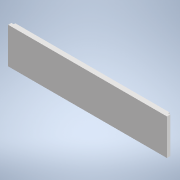
# Autodesk Inventor part: Arcade_FrontBottom
Saved by Autodesk Inventor 2022 (Build 260153000, 153)
## iProperties
Created: 2023-12-22
Part Number: Arcade_FrontBottom
Material: Generic
Document SubType Name: Modeling
Designer: Petr Černý
Density: 1 g/cm^3
Appearance: Default
Author: Petr Černý
Autodesk Inventor part; units mm, degrees
ref_plane "YZ Plane" through (0, 0, 0) normal (1, 0, 0) x (0, 1, 0)
ref_plane "XZ Plane" through (0, 0, 0) normal (0, 1, 0) x (-1, 0, 0)
ref_plane "XY Plane" through (0, 0, 0) normal (0, 0, 1) x (1, 0, 0)
sketch "Sketch1" plane through (0, 0, 0) normal (0, 0, 1) x (1, 0, 0)
  line L0 (-46.7038, 15.5679) -> (443.2962, 15.5679)
  line L1 (443.2962, 15.5679) -> (443.2962, -95.4321)
  line L2 (443.2962, -95.4321) -> (-46.7038, -95.4321)
  line L3 (-46.7038, -95.4321) -> (-46.7038, 15.5679)
  point P0 (0, 0)
  dimension "d0" = 490
  dimension "d1" = 111
  constraints: 8 end point, 2 parallel, 1 horizontal, 1 perpendicular
  measures "d0" distance of L1.end L2.end
  measures "d1" distance of L0.end L1.end
extrude "Extrusion1" add sketch "Sketch1" along normal blind 15
sketch "Sketch2" plane through (443.2962, -95.4321, 0) normal (1, 0, 0) x (0, 0, -1)
  line L0 (0, 0) -> (0, 111) projected
  line L1 (0, 111) -> (-5, 111)
  line L2 (-5, 111) -> (-5, 0)
  line L3 (-5, 0) -> (0, 0)
  line L4 (0, 0) -> (0, 111)
  point P0 (0, 95.4321)
  dimension "d4" = 5
  dimension "d5" = 111
  constraints: 8 end point, 2 parallel, 1 horizontal, 1 perpendicular
  measures "d4" distance of L3.end L2.end
  measures "d5" distance of L2.end L1.end
extrude "Extrusion2" cut sketch "Sketch2" against normal blind 7
sketch "Sketch3" plane through (-46.7038, -95.4321, 0) normal (-1, 0, 0) x (0, 0, 1)
  line L0 (0, 111) -> (0, 0) projected
  line L1 (0, 111) -> (5, 111)
  line L2 (5, 111) -> (5, 0)
  line L3 (5, 0) -> (0, 0)
  line L4 (0, 0) -> (0, 111)
  point P0 (0, 95.4321)
  dimension "d8" = 5
  dimension "d9" = 111
  constraints: 8 end point, 2 parallel, 1 horizontal, 1 perpendicular
  measures "d8" distance of L2.end L3.end
  measures "d9" distance of L1.end L2.end
extrude "Extrusion3" cut sketch "Sketch3" against normal blind 7
sketch "Sketch4" plane through (0, 0, 0) normal (0, 0, -1) x (-1, 0, 0)
  line L0 (-436.2962, 15.5679) -> (-436.2962, -95.4321) projected
  line L1 (-436.2962, 15.5679) -> (39.7038, 15.5679)
  line L2 (39.7038, 15.5679) -> (39.7038, 5.5679)
  line L3 (39.7038, 5.5679) -> (-436.2962, 5.5679)
  line L4 (-436.2962, 5.5679) -> (-436.2962, 15.5679)
  point P0 (0, 0)
  dimension "d12" = 476
  dimension "d13" = 10
  constraints: 8 end point, 2 parallel, 1 horizontal, 1 perpendicular
  measures "d12" distance of L2.end L3.end
  measures "d13" distance of L1.end L2.end
extrude "Extrusion4" cut sketch "Sketch4" against normal blind 5
body "Solid1"
